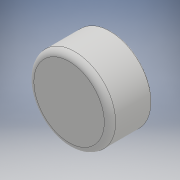
# Autodesk Inventor part: kork 32
Saved by Autodesk Inventor 2018 (Build 220112000, 112)
## iProperties
Created: 2018-06-16
Part Number: kork 32
Material: Generic
Document SubType Name: Modeling
Designer: dilan haddad
Density: 1 g/cm^3
Appearance: Default
Author: dilan haddad
Autodesk Inventor part; units mm, degrees
ref_plane "YZ Plane" through (0, 0, 0) normal (1, 0, 0) x (0, 1, 0)
ref_plane "XZ Plane" through (0, 0, 0) normal (0, 1, 0) x (-1, 0, 0)
ref_plane "XY Plane" through (0, 0, 0) normal (0, 0, 1) x (1, 0, 0)
sketch "Sketch1" plane through (0, 0, 0) normal (0, 1, 0) x (-1, 0, 0)
  circle A0 centre (0, 0) radius 10.75
  dimension "d0" = 21.5
  constraints: 1 centre point, 1 coincident
  measures "d0" diameter of A0
extrude "Extrusion1" add sketch "Sketch1" along normal blind 11
sketch "Sketch2" plane through (0, 11, 0) normal (0, 1, 0) x (1, 0, 0)
  circle A0 centre (0, 0) radius 10
  dimension "d3" = 20
  constraints: 1 centre point, 1 coincident
  measures "d3" diameter of A0
extrude "Extrusion2" cut sketch "Sketch2" against normal blind 10
fillet "Fillet1" radius 1.5 1 edges at (10.75, 0, 0)
fillet "Fillet2" radius 0.25 2 edges at (10.75, 11, 0) (-10, 11, 0)
thread "Thread1" size "M20x2.5" class "6H" standard "ANSI Metric M Profile" full length
body "Solid1"
